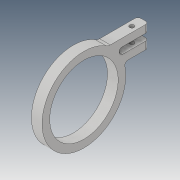
# Autodesk Inventor part: cameraBracket
Saved by Autodesk Inventor 2018 (Build 220112000, 112)
## iProperties
Created: 2019-11-23
Part Number: cameraBracket
Material: Generic
Document SubType Name: Modeling
Designer: anirudh
Density: 1 g/cm^3
Appearance: Default
Author: anirudh
Autodesk Inventor part; units mm, degrees
ref_plane "YZ Plane" through (0, 0, 0) normal (1, 0, 0) x (0, 1, 0)
ref_plane "XZ Plane" through (0, 0, 0) normal (0, 1, 0) x (-1, 0, 0)
ref_plane "XY Plane" through (0, 0, 0) normal (0, 0, 1) x (1, 0, 0)
sketch "Sketch1" plane through (0, 0, 0) normal (1, 0, 0) x (0, 1, 0)
  circle A0 centre (0, 0) radius 28.575
  line L0 (22.225, -26.9408) -> (22.225, -53.975)
  line L1 (22.225, -53.975) -> (28.575, -53.975)
  line L2 (28.575, -53.975) -> (28.575, -20.0805)
  line L3 (16.637, -53.975) -> (16.637, -30.7077)
  line L4 (16.637, -53.975) -> (10.287, -53.975)
  line L5 (10.287, -53.975) -> (10.287, -33.3756)
  arc A1 (28.575, -20.0805) -> (10.287, -33.3756) centre (0, 0) ccw
  arc A2 (16.637, -30.7077) -> (22.225, -26.9408) centre (0, 0) ccw
  dimension "d0" = 57.15
  dimension "d4" = 6.35
  dimension "d5" = 5.588
  dimension "d6" = 6.35
  constraints: 12 end point, 4 point on circle, 3 centre point, 2 coincident, 2 horizontal, 2 perpendicular
  measures "d0" diameter of A0
  measures "d4" distance of L0.end L1.end
  measures "d5" distance of L0.end L3.start
  measures "d6" distance of L3.start L4.end
extrude "Extrusion1" add sketch "Sketch1" along normal blind 8.89
sketch "Sketch2" plane through (0, 28.575, -20.0805) normal (0, 1, 0) x (1, 0, 0)
  line L0 (0, 33.8945) -> (8.89, 33.8945) projected
  line L1 (0, 33.8945) -> (8.89, 33.8945)
  line L2 (8.89, 6.8603) -> (8.89, 33.8945) projected
  line L3 (0, 33.8945) -> (8.89, 33.8945) projected
  circle A0 centre (4.445, 24.3695) radius 1.85
  point P0 (0, -20.0805)
  dimension "d23" = 3.7
  constraints: 2 end point, 1 centre point, 1 horizontal
  measures "d23" diameter of A0
fillet "Fillet1" radius 6.35 1 edges at (4.445, 28.575, -20.0805)
fillet "Fillet2" radius 2.54 1 edges at (4.445, 10.287, -33.3756)
fillet "Fillet3" radius 2.54 2 edges at (4.445, 22.225, -26.9408) (4.445, 16.637, -30.7077)
fillet "Fillet4" radius 2.54 4 edges at (8.89, 25.4, -53.975) (0, 25.4, -53.975) (0, 13.462, -53.975) (8.89, 13.462, -53.975)
extrude "Extrusion3" cut sketch "Sketch2" against normal blind 31.115
body "Solid1"
